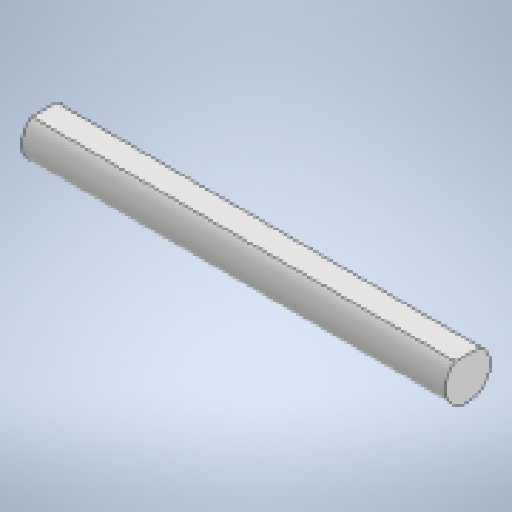
# Autodesk Inventor part: 2101-0006-0056
Saved by Autodesk Inventor 2023 (Build 270158000, 158)
## iProperties
Created: 2022-09-30
Part Number: 2101-0006-0056
Material: Generic
Document SubType Name: Modeling
Designer: deli
Density: 1 g/cm^3
Appearance: Default
Author: deli
Autodesk Inventor part; units mm, degrees
ref_plane "YZ Plane" through (0, 0, 0) normal (1, 0, 0) x (0, 1, 0)
ref_plane "XZ Plane" through (0, 0, 0) normal (0, 1, 0) x (-1, 0, 0)
ref_plane "XY Plane" through (0, 0, 0) normal (0, 0, 1) x (1, 0, 0)
sketch "Sketch1" plane through (0, 0, 0) normal (1, 0, 0) x (0, 1, 0)
  arc A0 (16.6744, 50.7127) -> (16.6744, 47.396) centre (14.1744, 49.0544) ccw
  line L0 (16.6744, 50.7127) -> (16.6744, 47.396)
  point P0 (0, 0)
  dimension "d0" = 6
  dimension "d1" = 2.5
  constraints: 2 end point, 2 point on circle, 1 centre point, 1 vertical
  measures "d0" diameter of A0
  measures "d1" distance from line of A0.centre L0
extrude "Extrusion1" add sketch "Sketch1" along normal blind 56
body "Solid1"
